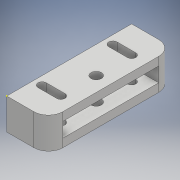
# Autodesk Inventor part: 3C_LiPoBatteryHolder_mountingBracket
Saved by Autodesk Inventor 2018 (Build 220112000, 112)
## iProperties
Created: 2019-07-06
Part Number: 3C_LiPoBatteryHolder_mountingBracket
Material: Generic
Document SubType Name: Modeling
Designer: Chris Taylor
Density: 1 g/cm^3
Appearance: Default
Author: Chris Taylor
Autodesk Inventor part; units mm, degrees
ref_plane "YZ Plane" through (0, 0, 0) normal (1, 0, 0) x (0, 1, 0)
ref_plane "XZ Plane" through (0, 0, 0) normal (0, 1, 0) x (-1, 0, 0)
ref_plane "XY Plane" through (0, 0, 0) normal (0, 0, 1) x (1, 0, 0)
sketch "Sketch1" plane through (0, 0, 0) normal (0, 0, 1) x (1, 0, 0)
  line L0 (0, 0) -> (20, 0)
  line L1 (20, 0) -> (20, 60)
  line L2 (20, 60) -> (0, 60)
  line L3 (0, 60) -> (0, 0)
  dimension "d0" = 20
  dimension "d1" = 60
  constraints: 8 end point, 2 parallel, 1 horizontal, 1 perpendicular
  measures "d0" distance of L2.end L1.end
  measures "d1" distance of L1.end L0.end
extrude "Extrusion1" add sketch "Sketch1" along normal blind 15
fillet "Fillet1" radius 7 2 edges at (20, 60, 7.5) (20, 0, 7.5)
sketch "Sketch2" plane through (0, 0, 15) normal (0, 0, 1) x (1, 0, 0)
  arc A0 (20, 53) -> (13, 60) centre (13, 53) ccw projected
  line L0 (13, 60) -> (13, 32.5)
  line L1 (13, 60) -> (13, 47)
  arc A1 (13, 0) -> (20, 7) centre (13, 7) ccw projected
  line L2 (13, 0) -> (13, 13)
  line L3 (13, 47) -> (4, 47) construction
  line L4 (13, 45) -> (4, 45)
  line L5 (4, 49) -> (13, 49)
  arc A2 (13, 45) -> (13, 49) centre (13, 47) ccw
  arc A3 (4, 49) -> (4, 45) centre (4, 47) ccw
  line L6 (13, 13) -> (4, 13) construction
  line L7 (13, 11) -> (4, 11)
  line L8 (4, 15) -> (13, 15)
  arc A4 (13, 11) -> (13, 15) centre (13, 13) ccw
  arc A5 (4, 15) -> (4, 11) centre (4, 13) ccw
  line L9 (13, 60) -> (0, 60) projected
  line L10 (13, 60) -> (13, 30)
  circle A6 centre (13, 30) radius 2.5
  point P0 (0, 0)
  point P1 (8.5, 47)
  point P2 (8.5, 13)
  dimension "d5" = 27.5
  dimension "d7" = 13
  dimension "d8" = 13
  dimension "d13" = 30
  dimension "d14" = 5
  constraints: 24 end point, 8 point on circle, 8 tangent, 5 centre point, 2 midpoint, 2 parallel, 2 perpendicular, 2 point on line, 2 vertical, 1 coincident
  measures "d5" distance of L0.start L0.end
  measures "d7" distance of L0.start L1.end
  measures "d8" distance of L2.start L2.end
  measures "d13" distance of L0.start L10.end
  measures "d14" diameter of A6
extrude "Extrusion2" cut sketch "Sketch2" against normal through all
sketch "Sketch3" plane through (20, 7, 0) normal (1, 0, 0) x (0, 0, -1)
  line L0 (-14, 0) -> (-14, 46)
  line L1 (-14, 0) -> (-6, 0)
  line L2 (-6, 0) -> (-6, 46)
  line L3 (-6, 46) -> (-14, 46)
  line L4 (-14, 46) -> (-14, 0)
  point P0 (0, -7)
  constraints: 10 end point, 2 parallel, 1 horizontal, 1 perpendicular
extrude "Extrusion3" cut sketch "Sketch3" against normal blind 20
sketch "Sketch4" plane through (0, 0, 15) normal (0, 0, 1) x (1, 0, 0)
  point P0 (0, 0)
sketch "Sketch5" plane through (0, 0, 15) normal (0, 0, 1) x (1, 0, 0)
  point P0 (0, 0)
sketch "Sketch6" plane through (20, 7, 14) normal (0, 0, -1) x (-1, 0, 0)
  line L0 (0, 46) -> (0, 0) projected
  line L1 (0, 0) -> (20, 0)
  line L2 (20, 0) -> (20, 46)
  line L3 (20, 46) -> (0, 46)
  line L4 (0, 46) -> (0, 0)
  point P0 (20, -7)
  constraints: 8 end point, 2 parallel, 1 horizontal, 1 perpendicular
extrude "Extrusion4" add sketch "Sketch6" along normal blind 3
sketch "Sketch7" plane through (0, 0, 15) normal (0, 0, 1) x (1, 0, 0)
  circle A0 centre (13, 30) radius 2.5
  point P0 (0, 0)
  constraints: 1 centre point
extrude "Extrusion5" cut sketch "Sketch7" against normal through all
sketch "Sketch8" plane through (0, 0, 15) normal (0, 0, 1) x (1, 0, 0)
  arc A0 (13, 11) -> (13, 15) centre (13, 13) ccw projected
  line L0 (13, 11) -> (4, 11) projected
  line L1 (13, 11) -> (4, 11)
  line L2 (4, 11) -> (4, 11)
  line L3 (4, 11) -> (13, 11)
  line L4 (13, 11) -> (13, 11)
  arc A1 (13, 45) -> (13, 49) centre (13, 47) ccw projected
  line L5 (4, 45) -> (13, 45) projected
  line L6 (13, 45) -> (13, 45)
  line L7 (13, 45) -> (4, 45)
  line L8 (4, 45) -> (4, 45)
  line L9 (4, 45) -> (13, 45)
  arc A2 (13, 45) -> (13, 49) centre (13, 47) ccw
  arc A3 (4, 49) -> (4, 45) centre (4, 47) ccw projected
  arc A4 (4, 49) -> (4, 45) centre (4, 47) ccw
  arc A5 (13, 11) -> (13, 15) centre (13, 13) ccw
  arc A6 (4, 15) -> (4, 11) centre (4, 13) ccw
  line L10 (4, 15) -> (13, 15) projected
  line L11 (4, 15) -> (13, 15)
  line L12 (4, 49) -> (13, 49) projected
  line L13 (4, 49) -> (13, 49)
  arc A7 (4, 49) -> (4, 45) centre (4, 47) ccw projected
  line L14 (13, 45) -> (4, 45)
  arc A8 (4, 15) -> (4, 11) centre (4, 13) ccw projected
  arc A9 (4, 15) -> (4, 15) centre (4, 13) ccw
  point P0 (0, 0)
  constraints: 22 end point, 8 point on circle, 7 equal length, 4 centre point, 3 coincident, 2 perpendicular, 1 tangent, 1 vertical alignment, 6 other
extrude "Extrusion6" cut sketch "Sketch8" against normal through all
sketch "Sketch9" plane through (20, 7, 6) normal (0, 0, 1) x (1, 0, 0)
  line L0 (0, 46) -> (-20, 46) projected
  arc A0 (-7, -7) -> (0, 0) centre (-7, 0) ccw projected
  line L1 (-20, 46) -> (0, 46)
  line L2 (0, 46) -> (0, 0)
  line L3 (0, 0) -> (-20, 0)
  line L4 (-20, 0) -> (-20, 46)
  point P0 (-20, -7)
  constraints: 8 end point, 2 parallel, 1 horizontal, 1 perpendicular
extrude "Extrusion7" cut sketch "Sketch9" against normal blind 2
body "Solid1"
